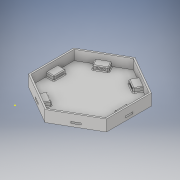
# Autodesk Inventor part: hexlight
Saved by Autodesk Inventor 2019 (Build 230136000, 136)
## iProperties
Created: 2019-03-04
Part Number: hexlight
Material: Generic
Document SubType Name: Modeling
Designer: Adam
Density: 1 g/cm^3
Appearance: Default
Author: Adam
Autodesk Inventor part; units mm, degrees
note: some values were not read from the file. Chosen so that the rebuilt part matches the saved one: direction of "Emboss1".
ref_plane "YZ Plane" through (0, 0, 0) normal (1, 0, 0) x (0, 1, 0)
ref_plane "XZ Plane" through (0, 0, 0) normal (0, 1, 0) x (-1, 0, 0)
sketch "Sketch1" plane through (0, 0, 0) normal (0, 1, 0) x (-1, 0, 0)
  line L0 (103.923, -30) -> (103.923, -90)
  line L1 (51.9615, -120) -> (0, -90)
  line L2 (0, -90) -> (0, -30)
  line L3 (0, -30) -> (51.9615, 0)
  line L4 (51.9615, 0) -> (103.923, -30)
  line L5 (103.923, -90) -> (51.9615, -120)
  point P0 (0, 0)
  dimension "d0" = 60
  dimension "d1" = 60
  dimension "d2" = 60
  dimension "d3" = 60
  dimension "d4" = 60
  dimension "d5" = 120
  dimension "d6" = 120
  dimension "d7" = 120
  dimension "d8" = 120
  dimension "d9" = 0
  dimension "d10" = 0
  constraints: 12 end point
  measures "d0" distance of L3.end L0.start
  measures "d1" distance of L2.end L3.end
  measures "d2" distance of L1.end L2.end
  measures "d3" distance of L1.start L1.end
  measures "d4" distance of L0.start L0.end
  measures "d5" angle of L4 L0
  measures "d6" angle of L3 L4
  measures "d7" angle of L2 L3
  measures "d8" angle of L1 L2
  measures "d9" distance from line of point (0, 0) L2
  measures "d10" vertical distance of point (0, 0) L3.end
extrude "Extrusion1" add sketch "Sketch1" along normal blind 15
sketch "Sketch2" plane through (0, 15, 0) normal (0, 1, 0) x (1, 0, 0)
  line L0 (-103.923, 90) -> (-103.923, 30) projected
  line L1 (-103.923, 30) -> (-51.9615, 0) projected
  line L2 (-103.923, 90) -> (-103.923, 30) projected
  line L3 (-103.923, 30) -> (-51.9615, 0) projected
  line L4 (-51.9615, 0) -> (0, 30) projected
  line L5 (0, 30) -> (0, 90) projected
  line L6 (0, 90) -> (-51.9615, 120) projected
  line L7 (-51.9615, 120) -> (-103.923, 90) projected
  line L8 (-51.9615, 2.3094) -> (-101.923, 31.1547)
  line L9 (-101.923, 31.1547) -> (-101.923, 88.8453)
  line L10 (0, 30) -> (0, 90) projected
  line L11 (0, 90) -> (-51.9615, 120) projected
  line L12 (-2, 31.1547) -> (-2, 88.8453)
  line L13 (-51.9615, 2.3094) -> (-2, 31.1547)
  line L14 (-51.9615, 117.6906) -> (-2, 88.8453)
  line L15 (-101.923, 88.8453) -> (-51.9615, 117.6906)
  point P0 (0, 0)
  dimension "d33" = 2
  dimension "d38" = 2
  constraints: 12 end point, 6 parallel, 1 vertical
  measures "d33" distance between parallel lines of L8 L1
  measures "d38" distance between parallel lines of L0 L9
extrude "Extrusion2" cut sketch "Sketch2" against normal blind 13 contours L8 L9 L15 L14 L12 L13
ref_plane "Work Plane1" through (0, -2549.525, 0) normal (0, -1, 0) x (1, 0, 0)
sketch "Sketch3" plane through (0, -2549.525, 0) normal (0, -1, 0) x (1, 0, 0)
  line L0 (-74.3693, -55.92) -> (-29.1273, -55.92) construction
  line L1 (-29.1273, -55.92) -> (-29.1273, -19.4796) construction
  line L2 (-29.1273, -19.4796) -> (-74.3693, -19.4796) construction
  line L3 (-74.3693, -19.4796) -> (-74.3693, -55.92) construction
  line L4 (-70.2662, -55.92) -> (-69.5538, -55.92)
  line L5 (-69.5538, -55.92) -> (-69.5538, -60.92)
  line L6 (-69.5538, -60.92) -> (-70.2662, -60.92)
  line L7 (-70.2662, -60.92) -> (-70.2662, -58.6744)
  line L8 (-70.2662, -58.6744) -> (-73.027, -58.6744)
  line L9 (-73.027, -58.6744) -> (-73.027, -60.92)
  line L10 (-73.027, -60.92) -> (-73.7395, -60.92)
  line L11 (-73.7395, -60.92) -> (-73.7395, -55.92)
  line L12 (-73.7395, -55.92) -> (-73.027, -55.92)
  line L13 (-73.027, -55.92) -> (-73.027, -58.0701)
  line L14 (-73.027, -58.0701) -> (-70.2662, -58.0701)
  line L15 (-70.2662, -58.0701) -> (-70.2662, -55.92)
  line L16 (-67.8975, -60.4607) -> (-66.0314, -60.4607)
  line L17 (-66.0314, -60.4607) -> (-66.0314, -60.92)
  line L18 (-66.0314, -60.92) -> (-68.439, -60.92)
  line L19 (-68.439, -60.92) -> (-68.439, -57.12)
  line L20 (-68.439, -57.12) -> (-66.0604, -57.12)
  line L21 (-66.0604, -57.12) -> (-66.0604, -57.5793)
  line L22 (-66.0604, -57.5793) -> (-67.8975, -57.5793)
  line L23 (-67.8975, -57.5793) -> (-67.8975, -58.7637)
  line L24 (-67.8975, -58.7637) -> (-66.2876, -58.7637)
  line L25 (-66.2876, -58.7637) -> (-66.3456, -59.2085)
  line L26 (-66.3456, -59.2085) -> (-67.8975, -59.2085)
  line L27 (-67.8975, -59.2085) -> (-67.8975, -60.4607)
  line L28 (-63.7108, -58.9426) -> (-62.4151, -60.92)
  line L29 (-62.4151, -60.92) -> (-63.0484, -60.92)
  line L30 (-63.0484, -60.92) -> (-64.0443, -59.3197)
  line L31 (-64.0443, -59.3197) -> (-65.0741, -60.92)
  line L32 (-65.0741, -60.92) -> (-65.6446, -60.92)
  line L33 (-65.6446, -60.92) -> (-64.3683, -58.9668)
  line L34 (-64.3683, -58.9668) -> (-65.5914, -57.12)
  line L35 (-65.5914, -57.12) -> (-64.9629, -57.12)
  line L36 (-64.9629, -57.12) -> (-64.0202, -58.5994)
  line L37 (-64.0202, -58.5994) -> (-63.0726, -57.12)
  line L38 (-63.0726, -57.12) -> (-62.5021, -57.12)
  line L39 (-62.5021, -57.12) -> (-63.7108, -58.9426)
  line L40 (-60.9713, -60.3029) -> (-58.5158, -60.3029)
  line L41 (-58.5158, -60.3029) -> (-58.5158, -60.92)
  line L42 (-58.5158, -60.92) -> (-61.6838, -60.92)
  line L43 (-61.6838, -60.92) -> (-61.6838, -55.92)
  line L44 (-61.6838, -55.92) -> (-60.9713, -55.92)
  line L45 (-60.9713, -55.92) -> (-60.9713, -60.3029)
  line L46 (-57.8973, -60.92) -> (-57.8973, -57.12)
  line L47 (-57.8973, -57.12) -> (-57.3558, -57.12)
  line L48 (-57.3558, -57.12) -> (-57.3558, -60.92)
  line L49 (-57.3558, -60.92) -> (-57.8973, -60.92)
  line L50 (-53.4349, -58.8121) -> (-53.4349, -60.6686)
  spline S0 degree 2 poles (-53.4349, -60.6686) (-53.783, -60.8329) (-54.3922, -60.9925) (-54.7934, -60.9925) knots 0 0 0 1 2 2 2
  spline S1 degree 2 poles (-54.7934, -60.9925) (-55.4219, -60.9925) (-56.2293, -60.4897) (-56.6064, -59.605) (-56.6064, -59.0248) knots 0 0 0 1 2 3 3 3
  spline S2 degree 2 poles (-56.6064, -59.0248) (-56.6064, -58.3431) (-56.1133, -57.4584) (-55.2914, -57.0475) (-54.7934, -57.0475) knots 0 0 0 1 2 3 3 3
  spline S3 degree 2 poles (-54.7934, -57.0475) (-54.426, -57.0475) (-53.8024, -57.2215) (-53.5268, -57.3955) knots 0 0 0 1 2 2 2
  line L51 (-53.5268, -57.3955) -> (-53.7637, -57.8017)
  spline S4 degree 2 poles (-53.7637, -57.8017) (-53.9667, -57.676) (-54.455, -57.5164) (-54.7548, -57.5164) knots 0 0 0 1 2 2 2
  spline S5 degree 2 poles (-54.7548, -57.5164) (-55.4171, -57.5164) (-56.0311, -58.3093) (-56.0311, -59.0006) knots 0 0 0 1 2 2 2
  spline S6 degree 2 poles (-56.0311, -59.0006) (-56.0311, -59.7307) (-55.4461, -60.5235) (-54.7838, -60.5235) knots 0 0 0 1 2 2 2
  spline S7 degree 2 poles (-54.7838, -60.5235) (-54.3728, -60.5235) (-53.9764, -60.3737) knots 0 0 0 1 1 1
  line L52 (-53.9764, -60.3737) -> (-53.9764, -59.2714)
  line L53 (-53.9764, -59.2714) -> (-54.9482, -59.2714)
  line L54 (-54.9482, -59.2714) -> (-54.8901, -58.8121)
  line L55 (-54.8901, -58.8121) -> (-53.4349, -58.8121)
  line L56 (-49.983, -57.12) -> (-49.4415, -57.12)
  line L57 (-49.4415, -57.12) -> (-49.4415, -60.92)
  line L58 (-49.4415, -60.92) -> (-49.983, -60.92)
  line L59 (-49.983, -60.92) -> (-49.983, -59.2134)
  line L60 (-49.983, -59.2134) -> (-52.0812, -59.2134)
  line L61 (-52.0812, -59.2134) -> (-52.0812, -60.92)
  line L62 (-52.0812, -60.92) -> (-52.6227, -60.92)
  line L63 (-52.6227, -60.92) -> (-52.6227, -57.12)
  line L64 (-52.6227, -57.12) -> (-52.0812, -57.12)
  line L65 (-52.0812, -57.12) -> (-52.0812, -58.7541)
  line L66 (-52.0812, -58.7541) -> (-49.983, -58.7541)
  line L67 (-49.983, -58.7541) -> (-49.983, -57.12)
  line L68 (-45.6802, -57.12) -> (-45.6802, -57.5889)
  line L69 (-45.6802, -57.5889) -> (-46.9904, -57.5889)
  line L70 (-46.9904, -57.5889) -> (-46.9904, -60.92)
  line L71 (-46.9904, -60.92) -> (-47.5319, -60.92)
  line L72 (-47.5319, -60.92) -> (-47.5319, -57.5889)
  line L73 (-47.5319, -57.5889) -> (-48.8517, -57.5889)
  line L74 (-48.8517, -57.5889) -> (-48.8517, -57.12)
  line L75 (-48.8517, -57.12) -> (-45.6802, -57.12)
  line L76 (-41.1006, -57.92) -> (-41.1006, -60.92)
  line L77 (-41.1006, -60.92) -> (-41.3601, -60.92)
  line L78 (-41.3601, -60.92) -> (-41.3601, -58.3246)
  spline S8 degree 2 poles (-41.3601, -58.3246) (-41.4288, -58.481) (-41.5281, -58.6719) knots 0 0 0 1 1 1
  line L79 (-41.5281, -58.6719) -> (-42.4326, -60.3894)
  line L80 (-42.4326, -60.3894) -> (-42.696, -60.3894)
  line L81 (-42.696, -60.3894) -> (-43.5853, -58.6719)
  line L82 (-43.5853, -58.6719) -> (-43.6311, -58.5765)
  spline S9 degree 2 poles (-43.6311, -58.5765) (-43.7074, -58.4391) (-43.7532, -58.336) knots 0 0 0 1 1 1
  line L83 (-43.7532, -58.336) -> (-43.7532, -60.92)
  line L84 (-43.7532, -60.92) -> (-44.0128, -60.92)
  line L85 (-44.0128, -60.92) -> (-44.0128, -57.92)
  line L86 (-44.0128, -57.92) -> (-43.7113, -57.92)
  line L87 (-43.7113, -57.92) -> (-42.7952, -59.6719)
  line L88 (-42.7952, -59.6719) -> (-42.7303, -59.8017)
  spline S10 degree 2 poles (-42.7303, -59.8017) (-42.6044, -60.0421) (-42.5586, -60.1528) knots 0 0 0 1 1 1
  spline S11 degree 2 poles (-42.5586, -60.1528) (-42.5166, -60.0574) (-42.3906, -59.8017) (-42.3219, -59.6719) knots 0 0 0 1 2 2 2
  line L89 (-42.3219, -59.6719) -> (-41.3868, -57.92)
  line L90 (-41.3868, -57.92) -> (-41.1006, -57.92)
  line L91 (-39.0891, -57.92) -> (-37.8983, -60.8971)
  line L92 (-37.8983, -60.8971) -> (-37.8983, -60.92)
  line L93 (-37.8983, -60.92) -> (-38.1655, -60.92)
  line L94 (-38.1655, -60.92) -> (-38.5357, -59.981)
  line L95 (-38.5357, -59.981) -> (-39.9326, -59.981)
  line L96 (-39.9326, -59.981) -> (-40.2952, -60.92)
  line L97 (-40.2952, -60.92) -> (-40.5471, -60.92)
  line L98 (-40.5471, -60.92) -> (-40.5471, -60.8971)
  line L99 (-40.5471, -60.8971) -> (-39.3677, -57.92)
  line L100 (-39.3677, -57.92) -> (-39.0891, -57.92)
  line L101 (-39.8448, -59.7635) -> (-38.6197, -59.7635)
  line L102 (-38.6197, -59.7635) -> (-39.2303, -58.1986)
  line L103 (-39.2303, -58.1986) -> (-39.8448, -59.7635)
  line L104 (-35.2723, -60.8971) -> (-35.2723, -60.92)
  line L105 (-35.2723, -60.92) -> (-35.5624, -60.92)
  line L106 (-35.5624, -60.92) -> (-36.5128, -59.6757)
  line L107 (-36.5128, -59.6757) -> (-37.0929, -59.6757)
  line L108 (-37.0929, -59.6757) -> (-37.0929, -60.92)
  line L109 (-37.0929, -60.92) -> (-37.3525, -60.92)
  line L110 (-37.3525, -60.92) -> (-37.3525, -57.92)
  line L111 (-37.3525, -57.92) -> (-36.4784, -57.92)
  spline S12 degree 2 poles (-36.4784, -57.92) (-36.1502, -57.92) (-35.6769, -58.1299) (-35.4288, -58.5116) (-35.4288, -58.7711) knots 0 0 0 1 2 3 3 3
  spline S13 degree 2 poles (-35.4288, -58.7711) (-35.4288, -59.0001) (-35.6082, -59.3665) (-35.9708, -59.6146) (-36.2342, -59.6566) knots 0 0 0 1 2 3 3 3
  line L112 (-36.2342, -59.6566) -> (-35.2723, -60.8971)
  line L113 (-37.0929, -59.4581) -> (-36.4861, -59.4581)
  spline S14 degree 2 poles (-36.4861, -59.4581) (-36.0891, -59.4581) (-35.6884, -59.0955) (-35.6884, -58.7902) knots 0 0 0 1 2 2 2
  spline S15 degree 2 poles (-35.6884, -58.7902) (-35.6884, -58.4849) (-36.0891, -58.1413) (-36.4861, -58.1413) knots 0 0 0 1 2 2 2
  line L114 (-36.4861, -58.1413) -> (-37.0929, -58.1413)
  line L115 (-37.0929, -58.1413) -> (-37.0929, -59.4581)
  line L116 (-34.1616, -59.3551) -> (-32.654, -60.8971)
  line L117 (-32.654, -60.8971) -> (-32.654, -60.92)
  line L118 (-32.654, -60.92) -> (-32.9632, -60.92)
  line L119 (-32.9632, -60.92) -> (-34.467, -59.3818)
  line L120 (-34.467, -59.3818) -> (-34.467, -60.92)
  line L121 (-34.467, -60.92) -> (-34.7265, -60.92)
  line L122 (-34.7265, -60.92) -> (-34.7265, -57.92)
  line L123 (-34.7265, -57.92) -> (-34.467, -57.92)
  line L124 (-34.467, -57.92) -> (-34.467, -59.3475)
  line L125 (-34.467, -59.3475) -> (-33.0242, -57.92)
  line L126 (-33.0242, -57.92) -> (-32.7342, -57.92)
  line L127 (-32.7342, -57.92) -> (-32.7342, -57.9429)
  line L128 (-32.7342, -57.9429) -> (-34.1616, -59.3551)
  line L129 (-30.9899, -60.92) -> (-30.9899, -57.92)
  line L130 (-30.9899, -57.92) -> (-30.7303, -57.92)
  line L131 (-30.7303, -57.92) -> (-30.7303, -60.92)
  line L132 (-30.7303, -60.92) -> (-30.9899, -60.92)
  line L133 (-29.8372, -60.92) -> (-29.8372, -57.92)
  line L134 (-29.8372, -57.92) -> (-29.5777, -57.92)
  line L135 (-29.5777, -57.92) -> (-29.5777, -60.92)
  line L136 (-29.5777, -60.92) -> (-29.8372, -60.92)
  point P0 (0, 0)
  constraints: 2 other
emboss "Emboss1" sketch "Sketch3" operation cut depth 1 direction (0, 1, 0)
sketch "Sketch4" plane through (-101.923, 15, -31.1547) normal (1, 0, 0) x (0, 0, -1)
  line L0 (36.5602, -13) -> (20.5602, -13)
  line L1 (20.5602, -13) -> (20.5602, -7.5)
  line L2 (20.5602, -7.5) -> (36.5602, -7.5)
  line L3 (36.5602, -7.5) -> (36.5602, -13)
  line L4 (0, -13) -> (57.6906, -13) projected
  line L5 (0, 0) -> (0, -13) projected
  point P0 (-31.1547, -15)
  dimension "d45" = 16
  dimension "d46" = 5.5
  dimension "d47" = 0
  dimension "d48" = 20.5602
  constraints: 8 end point, 2 parallel, 1 horizontal, 1 perpendicular
  measures "d45" distance of L1.end L2.end
  measures "d46" distance of L0.end L1.end
  measures "d47" distance between parallel lines of L4 L0
  measures "d48" distance between parallel lines of L5 L1
extrude "Extrusion3" add sketch "Sketch4" along normal blind 10
fillet "Fillet1" radius 1 8 edges at (-91.923, 7.5, -59.7149) (-96.923, 7.5, -51.7149) (-96.923, 7.5, -67.7149) (-91.923, 2, -59.7149) (-91.923, 4.75, -51.7149) (-91.923, 4.75, -67.7149) (-96.923, 2, -67.7149) (-96.923, 2, -51.7149)
sketch "Sketch5" plane through (-91.923, 15, -31.1547) normal (1, 0, 0) x (0, 0, -1)
  point P0 (-31.1547, -15)
sketch "Sketch6" plane through (-91.923, 15, -31.1547) normal (1, 0, 0) x (0, 0, -1)
  line L0 (21.5602, -8.5) -> (35.5602, -8.5) projected
  line L1 (21.5602, -12) -> (21.5602, -8.5) projected
  point P0 (-31.1547, -15)
  point P1 (24.8852, -10.25)
  point P2 (27.4252, -10.25)
  point P3 (29.9652, -10.25)
  point P4 (32.5052, -10.25)
  dimension "d52" = 1.75
  dimension "d53" = 3.325
  dimension "d54" = 0
  dimension "d55" = 0
  dimension "d56" = 0
  dimension "d57" = 2.54
  dimension "d58" = 2.54
  dimension "d59" = 2.54
  measures "d52" distance from line of L0 point (24.885, -10.25)
  measures "d53" distance from line of L1 point (24.885, -10.25)
  measures "d54" vertical distance of point (24.885, -10.25) point (27.425, -10.25)
  measures "d55" vertical distance of point (27.425, -10.25) point (29.965, -10.25)
  measures "d56" vertical distance of point (29.965, -10.25) point (32.505, -10.25)
  measures "d57" distance of point (24.885, -10.25) point (27.425, -10.25)
  measures "d58" distance of point (27.425, -10.25) point (29.965, -10.25)
  measures "d59" distance of point (29.965, -10.25) point (32.505, -10.25)
hole "Hole1" at (-91.923, 4.75, -56.0399) at (-91.923, 4.75, -58.5799) at (-91.923, 4.75, -61.1199) at (-91.923, 4.75, -63.6599) direction (-1, 0, 0) diameter 2 end through all
sketch "Sketch7" plane through (-103.923, 0, -90) normal (-1, 0, 0) x (0, 0, 1)
  circle A0 centre (33.9601, 4.75) radius 1 construction
  line L0 (1.1547, 15) -> (58.8453, 15) projected
  line L1 (1.1547, 15) -> (1.1547, 2) projected
  line L2 (1.1547, 2) -> (58.8453, 2) projected
  line L3 (58.8453, 15) -> (58.8453, 2) projected
  line L4 (25.1501, 5.85) -> (25.1501, 3.65)
  line L5 (25.1501, 3.65) -> (35.1501, 3.65)
  line L6 (35.1501, 3.65) -> (35.1501, 5.85)
  line L7 (35.1501, 5.85) -> (25.1501, 5.85)
  point P0 (90, 0)
  point P1 (23.2851, 3)
  point P2 (37.2851, 3)
  point P3 (37.2851, 6.5)
  dimension "d74" = 2.2
  dimension "d75" = 10
  dimension "d76" = 1.1
  dimension "d77" = 1.19
  constraints: 8 end point, 3 perpendicular, 1 vertical
  measures "d74" distance of L4.start L4.end
  measures "d75" distance of L6.end L4.start
  measures "d76" distance from line of A0.centre L7
  measures "d77" distance from line of L6 A0.centre
extrude "Extrusion4" cut sketch "Sketch7" against normal blind 10 contours L7 L6 L5 L4
sketch "Sketch8" plane through (0, 2, 0) normal (0, 1, 0) x (1, 0, 0)
  line L0 (-51.9615, 0) -> (0, 30) projected
  line L1 (-103.923, 90) -> (-103.923, 30) projected
  point P0 (0, 0)
  point P1 (-51.9615, 60)
  dimension "d80" = 0
  dimension "d81" = 30
  measures "d80" horizontal distance of L0.start point (-51.962, 60)
  measures "d81" vertical distance of L1.start point (-51.962, 60)
pattern_circular "Circular Pattern1" count 6 over 360 about axis through (-51.9615, 2, -60) along (0, 1, 0) of "Extrusion3", "Hole1", "Extrusion4", "Fillet1"
body "Solid1"
